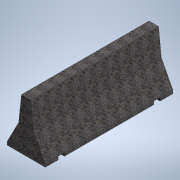
# Autodesk Inventor part: Jersey Curb
Saved by Autodesk Inventor 2022 (Build 260153000, 153)
## iProperties
Created: 2021-11-04
Part Number: Jersey Curb
Material: Concrete
Document SubType Name: Modeling
Designer: kibandi
Density: 2.40731 g/cm^3
Appearance: Exposed Aggregate - Coarse
Mass: 700737 g
Surface Area: 75182.7 cm^2
Volume: 291087 cm^3
Author: kibandi
Autodesk Inventor part; units mm, degrees
ref_plane "YZ Plane" through (0, 0, 0) normal (1, 0, 0) x (0, 1, 0)
ref_plane "XZ Plane" through (0, 0, 0) normal (0, 1, 0) x (-1, 0, 0)
ref_plane "XY Plane" through (0, 0, 0) normal (0, 0, 1) x (1, 0, 0)
sketch "Sketch1" plane through (0, 0, 0) normal (0, 0, 1) x (1, 0, 0)
  line L0 (0, 0) -> (0, 800) construction
  line L1 (0, 800) -> (-75, 800)
  line L2 (-300, 0) -> (-300, 50)
  line L3 (-75, 800) -> (-118.3113, 400)
  line L4 (-118.3113, 400) -> (-300, 50)
  line L5 (0, 800) -> (75, 800)
  line L6 (300, 0) -> (300, 50)
  line L7 (75, 800) -> (118.3113, 400)
  line L8 (118.3113, 400) -> (300, 50)
  line L9 (300, 0) -> (-300, 0)
  dimension "d28" = 800
  constraints: 20 end point, 4 symmetric about line, 1 horizontal, 1 vertical
  measures "d28" distance of L0.start L0.end
extrude "Extrusion1" add sketch "Sketch1" along normal mid plane 2000
sketch "Sketch5" plane through (-300, 0, 1000) normal (0, -1, 0) x (1, 0, 0)
  line L0 (0, -2000) -> (181.6887, -2000) projected
  line L1 (0, -2000) -> (0, 0) projected
  line L2 (100, -1900) -> (100, -100)
  line L3 (181.6887, -2000) -> (181.6887, 0) projected
  line L4 (100, -1900) -> (500, -1900)
  line L5 (600, -2000) -> (600, 0) projected
  line L6 (500, -1900) -> (500, -100)
  line L7 (500, -100) -> (100, -100)
  point P0 (300, -1000)
  dimension "d35" = 1800
  constraints: 8 end point, 1 horizontal, 1 parallel, 1 perpendicular
  measures "d35" distance of L4.end L6.end
extrude "Extrusion5" cut sketch "Sketch5" against normal blind 200
chamfer "Chamfer1" distance 130 angle 45 2 edges at (200, 200, 0) (-200, 200, 0)
sketch "Sketch6" plane through (-300, 200, 1000) normal (0, -1, 0) x (1, 0, 0)
  line L0 (370, -100) -> (370, -1900) projected
  line L1 (370, -100) -> (370, -1900)
  line L2 (230, -1900) -> (230, -100) projected
  line L3 (370, -1900) -> (230, -1900)
  line L4 (230, -1900) -> (230, -100)
  line L5 (230, -100) -> (370, -100)
  point P0 (300, -1000)
  constraints: 8 end point, 3 perpendicular, 1 collinear
extrude "Extrusion6" cut sketch "Sketch6" against normal blind 400
sketch "Sketch7" plane through (200, 0, -900) normal (-1, 0, 0) x (0, 0, 1)
  line L0 (0, 0) -> (0, 70) projected
  line L1 (0, 0) -> (100, 0)
  line L2 (1800, 0) -> (0, 0) projected
  line L3 (100, 0) -> (100, 50)
  line L4 (100, 50) -> (200, 50)
  line L5 (200, 50) -> (200, 0)
  line L6 (200, 0) -> (100, 0)
  line L7 (1800, 0) -> (1700, 0)
  line L8 (1700, 0) -> (1700, 50)
  line L9 (1700, 50) -> (1600, 50)
  line L10 (1600, 50) -> (1600, 0)
  line L11 (1600, 0) -> (1700, 0)
  point P0 (900, 0)
  point P1 (200, 0)
  dimension "d43" = 100
  dimension "d44" = 50
  dimension "d45" = 100
  dimension "d46" = 50
  dimension "d47" = 100
  dimension "d48" = 50
  dimension "d49" = 100
  dimension "d50" = 50
  constraints: 20 end point, 4 perpendicular, 4 point on line, 1 collinear
  measures "d43" distance of L0.start L1.end
  measures "d44" distance of L1.end L3.end
  measures "d45" distance of L3.end L4.end
  measures "d46" distance of L4.end L5.end
  measures "d47" distance of L2.start L7.end
  measures "d48" distance of L7.end L8.end
  measures "d49" distance of L8.end L9.end
  measures "d50" distance of L9.end L10.end
sketch "Sketch8" plane through (-200, 0, 900) normal (1, 0, 0) x (0, 0, -1)
  line L0 (1800, 0) -> (0, 0) projected
  line L1 (1800, 0) -> (1700, 0)
  line L2 (1700, 0) -> (1700, 50)
  line L3 (1700, 50) -> (1600, 50)
  line L4 (1600, 50) -> (1600, 0)
  line L5 (0, 0) -> (100, 0)
  line L6 (100, 0) -> (100, 50)
  line L7 (100, 50) -> (200, 50)
  line L8 (200, 50) -> (200, 0)
  line L9 (200, 0) -> (100, 0)
  point P0 (900, 0)
  dimension "d55" = 100
  dimension "d56" = 50
  dimension "d57" = 100
  dimension "d58" = 50
  dimension "d59" = 100
  dimension "d60" = 50
  dimension "d61" = 100
  dimension "d62" = 50
  constraints: 18 end point, 4 perpendicular, 4 point on line, 1 collinear
  measures "d55" distance of L0.start L1.end
  measures "d56" distance of L1.end L2.end
  measures "d57" distance of L2.end L3.end
  measures "d58" distance of L3.end L4.end
  measures "d59" distance of L0.end L5.end
  measures "d60" distance of L5.end L6.end
  measures "d61" distance of L6.end L7.end
  measures "d62" distance of L7.end L8.end
extrude "Extrusion7" cut sketch "Sketch8" against normal blind 100
extrude "Extrusion8" cut sketch "Sketch7" against normal blind 100
body "Solid1"
